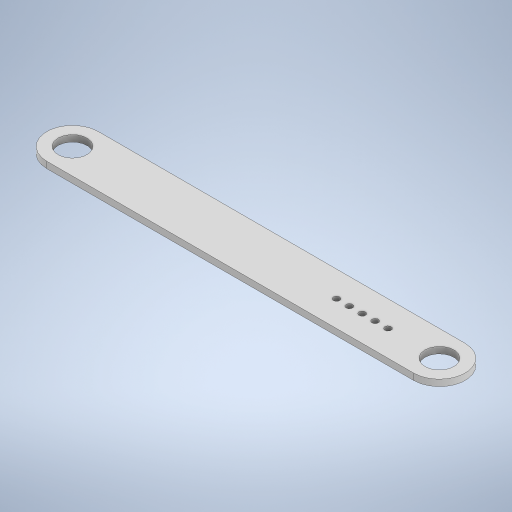
# Autodesk Inventor part: 4-bar intake (14.258) bar
Saved by Autodesk Inventor 2023 (Build 270158030, 158C)
## iProperties
Created: 2022-07-18
Part Number: 4-bar intake (14.258) bar
Material: Generic
Document SubType Name: Modeling
Designer: kt1040502
Density: 1 g/cm^3
Appearance: Default
Author: kt1040502
Autodesk Inventor part; units mm, degrees
ref_plane "YZ Plane" through (0, 0, 0) normal (1, 0, 0) x (0, 1, 0)
ref_plane "XZ Plane" through (0, 0, 0) normal (0, 1, 0) x (-1, 0, 0)
ref_plane "XY Plane" through (0, 0, 0) normal (0, 0, 1) x (1, 0, 0)
sketch "Sketch1" plane through (0, 0, 0) normal (0, 1, 0) x (-1, 0, 0)
  line L0 (0, 0) -> (-362.1532, 0)
  line L1 (0, 0) -> (-362.1532, 0) construction
  line L2 (0, 0) -> (-362.1532, 0) construction
  line L3 (0, 25.4) -> (-362.1532, 25.4)
  line L4 (-362.1532, -25.4) -> (0, -25.4)
  arc A0 (0, -25.4) -> (0, 25.4) centre (0, 0) ccw
  arc A1 (-362.1532, 25.4) -> (-362.1532, -25.4) centre (-362.1532, 0) ccw
  circle A2 centre (0, 0) radius 14.2875
  circle A3 centre (-362.1532, 0) radius 14.2875
  circle A4 centre (-311.3532, 0) radius 3.175
  circle A5 centre (-298.6532, 0) radius 3.175
  circle A6 centre (-285.9532, 0) radius 3.175
  circle A7 centre (-273.2532, 0) radius 3.175
  circle A8 centre (-260.5532, 0) radius 3.175
  point P0 (-181.0766, 0)
  point P1 (-181.0766, 0)
  dimension "d0" = 362.1532
  dimension "d8" = 50.8
  dimension "d9" = 28.575
  dimension "d10" = 28.575
  dimension "d11" = 6.35
  dimension "d12" = 50.8
  dimension "d13" = 6.35
  dimension "d14" = 6.35
  dimension "d15" = 6.35
  dimension "d16" = 6.35
  dimension "d17" = 12.7
  dimension "d18" = 12.7
  dimension "d19" = 12.7
  dimension "d20" = 12.7
  constraints: 14 end point, 9 centre point, 5 point on line, 4 point on circle, 4 tangent, 3 equal length, 2 coincident, 2 midpoint, 1 horizontal
  measures "d0" distance of L0.start L0.end
  measures "d8" diameter of A1
  measures "d9" diameter of A2
  measures "d10" diameter of A3
  measures "d11" diameter of A4
  measures "d12" distance of L0.end A4.centre
  measures "d13" diameter of A5
  measures "d14" diameter of A6
  measures "d15" diameter of A7
  measures "d16" diameter of A8
  measures "d17" distance of A4.centre A5.centre
  measures "d18" distance of A5.centre A6.centre
  measures "d19" distance of A6.centre A7.centre
  measures "d20" distance of A7.centre A8.centre
extrude "Extrusion1" add sketch "Sketch1" along normal blind 6.35
body "Solid1"
